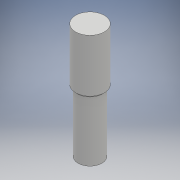
# Autodesk Inventor part: コガネイ_BDA16x5(円柱)
Saved by Autodesk Inventor 2018 (Build 220112000, 112)
## iProperties
Created: 2018-04-23
Part Number: コガネイ_BDA16x5(円柱)
Material: 一般
Document SubType Name: Modeling
Designer: Take
Density: 1 g/cm^3
Appearance: 既定
Author: Take
Autodesk Inventor part; units mm, degrees
ref_plane "YZ Plane" through (0, 0, 0) normal (1, 0, 0) x (0, 1, 0)
ref_plane "XZ Plane" through (0, 0, 0) normal (0, 1, 0) x (-1, 0, 0)
ref_plane "XY Plane" through (0, 0, 0) normal (0, 0, 1) x (1, 0, 0)
sketch "スケッチ1" plane through (0, 0, 0) normal (0, 1, 0) x (-1, 0, 0)
  line L0 (0, 0) -> (3, 0)
  line L1 (3, 0) -> (3, -11)
  line L2 (2.5, -11.5) -> (3, -11)
  line L3 (2.5, -11.5) -> (2.5, -12.5)
  line L4 (2.5, -12.5) -> (2.5, -24)
  line L5 (2.5, -24) -> (0, -24)
  line L6 (0, -24) -> (0, 0)
  point P0 (2.5, -11)
  dimension "d1" = 3
  dimension "d2" = 11
  dimension "d3" = 0.5
  dimension "d4" = 0.5
  dimension "d5" = 1
  dimension "d6" = 11.5
  constraints: 14 end point, 3 perpendicular, 2 vertical, 1 horizontal
  measures "d1" distance of L0.start L0.end
  measures "d2" distance of L0.end L1.end
  measures "d3" distance of L1.end point (2.5, -11)
  measures "d4" distance of L2.start point (2.5, -11)
  measures "d5" distance of L2.start L3.end
  measures "d6" distance of L3.end L4.end
revolve "回転1" add sketch "スケッチ1" angle 360 about axis through (0, 0, -24) along (0, 0, 1)
